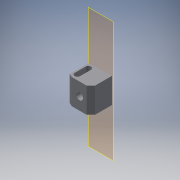
# Autodesk Inventor part: kinect_fixt
Saved by Autodesk Inventor 2019 (Build 230136000, 136)
## iProperties
Created: 2024-05-02
Part Number: kinect_fixt
Material: Generisch
Document SubType Name: Modeling
Designer: nic
Density: 1 g/cm^3
Appearance: Vorgabe
Author: nic
Autodesk Inventor part; units mm, degrees
ref_plane "YZ Plane" through (0, 0, 0) normal (1, 0, 0) x (0, 1, 0)
ref_plane "XZ Plane" through (0, 0, 0) normal (0, 1, 0) x (-1, 0, 0)
ref_plane "XY Plane" through (0, 0, 0) normal (0, 0, 1) x (1, 0, 0)
ref_plane "Arbeitsebene1" through (0, 0, 0) normal (0, 0, 1) x (1, 0, 0)
sketch "Skizze1" plane through (0, 0, 0) normal (0, 0, 1) x (1, 0, 0)
  circle A0 centre (-13.5, 65) radius 3 construction
  circle A1 centre (-13.5, 65) radius 3 construction
  line L0 (0, 130) -> (0, 0) construction
  line L1 (0, 130) -> (-27, 130) construction
  line L2 (-27, 0) -> (-27, 130) construction
  line L3 (0, 0) -> (-27, 0) construction
  line L4 (-27, 80) -> (0, 80)
  line L5 (0, 80) -> (0, 50)
  line L6 (0, 50) -> (-27, 50)
  line L7 (-27, 50) -> (-27, 80)
  line L8 (-27, 80) -> (0, 50) construction
  line L9 (0, 80) -> (-27, 50) construction
  dimension "d0" = 30
  constraints: 12 end point, 2 midpoint, 2 parallel, 1 horizontal, 1 perpendicular, 1 point on line
  measures "d0" distance of L4.end L5.end
extrude "Extrusion1" add sketch "Skizze1" along normal blind 25
sketch "Skizze2" plane through (0, 0, 25) normal (0, 0, 1) x (1, 0, 0)
  circle A0 centre (-13.5, 65) radius 3 projected
  circle A1 centre (-13.5, 65) radius 4.15
  point P0 (0, 0)
  dimension "d3" = 8.3
  constraints: 1 centre point, 1 coincident
  measures "d3" diameter of A1
extrude "Extrusion2" cut sketch "Skizze2" against normal through all contours A0 | A1
sketch "Skizze3" plane through (-27, 80, 0) normal (0, 1, 0) x (1, 0, 0)
  line L0 (0, 0) -> (0, -25) projected
  line L1 (0, 0) -> (5.0639, 0)
  line L2 (5.0639, 0) -> (5.0639, -24.302)
  line L3 (5.0639, -24.302) -> (0, -24.302)
  line L4 (0, -24.302) -> (0, 0)
  circle A0 centre (5.0639, -18.8642) radius 3.15
  circle A1 centre (5.0639, -8.0952) radius 3.15
  circle A2 centre (5.0639, -12.5) radius 3.25
  point P0 (27, 0)
  dimension "d6" = 6.3
  dimension "d7" = 6.3
  dimension "d10" = 6.5
  constraints: 8 end point, 3 centre point, 3 point on line, 2 parallel, 1 horizontal, 1 perpendicular
  measures "d6" diameter of A0
  measures "d7" diameter of A1
  measures "d10" diameter of A2
extrude "Extrusion4" cut sketch "Skizze3" against normal through all contours A2 A1 L2 | L2 A1 A2 | A1 L2 A0 A2 | A2 A0 L2 | L2 A0 A2 | A1 A2 A0 L2 picked at (5.2798, -10.5577) picked at (4.848, -10.5577) picked at (5.0263, -15.7268) picked at (5.1015, -15.7268)
sketch "Skizze4" plane through (-27, 80, 0) normal (0, 1, 0) x (1, 0, 0)
  line L0 (0, -25) -> (27, -25) projected
  line L1 (0, -25) -> (-134.4779, 33.9504) construction
  line L2 (0, 0) -> (0, -25) projected
  line L3 (0, -25) -> (4.3797, -25)
  line L4 (0, -23.0801) -> (0, -25)
  line L5 (4.3797, -25) -> (0, -23.0801)
  line L6 (4.3797, -25) -> (0, -25)
  point P0 (27, 0)
  constraints: 10 end point, 1 collinear, 1 horizontal
extrude "Extrusion5" cut sketch "Skizze4" against normal through all
chamfer "Fase1" distance 5 angle 45 1 edges at (0, 65, 25)
sketch "Skizze5" plane through (-27, 50, 0) normal (0, -1, 0) x (1, 0, 0)
  circle A0 centre (5.0639, 12.5) radius 3.25 construction
  line L0 (5.0639, 18.9193) -> (5.0639, 6.0807) construction
  line L1 (1.812, 18.9193) -> (1.812, 6.0807)
  line L2 (8.3158, 6.0807) -> (8.3158, 18.9193)
  arc A1 (8.3158, 18.9193) -> (1.812, 18.9193) centre (5.0639, 18.9193) ccw
  arc A2 (1.812, 6.0807) -> (8.3158, 6.0807) centre (5.0639, 6.0807) ccw
  point P0 (27, 0)
  constraints: 8 end point, 4 point on circle, 4 tangent, 2 centre point, 1 midpoint, 1 parallel, 1 vertical
extrude "Extrusion6" cut sketch "Skizze5" against normal through all
